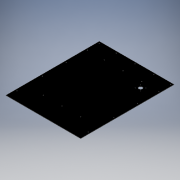
# Autodesk Inventor part: Side Cladding
Saved by Autodesk Inventor 2017.3 (Build 213256000, 256)
## iProperties
Created: 2018-10-13
Part Number: Side Cladding
Material: Aluminum 6061
Document SubType Name: Sheet Metal
Designer: Ax
Density: 2.7 g/cm^3
Sheet Metal Rule: Default_mm
Appearance: Anodized - Black
Author: Ax
Autodesk Inventor part; units mm, degrees
ref_plane "YZ Plane" through (0, 0, 0) normal (1, 0, 0) x (0, 1, 0)
ref_plane "XZ Plane" through (0, 0, 0) normal (0, 1, 0) x (-1, 0, 0)
ref_plane "XY Plane" through (0, 0, 0) normal (0, 0, 1) x (1, 0, 0)
sketch "Sketch1" plane through (0, 0, 0) normal (0, 0, 1) x (1, 0, 0)
  line L0 (-220, -275) -> (220, -275)
  line L1 (220, -275) -> (220, 275)
  line L2 (220, 275) -> (-220, 275)
  line L3 (-220, 275) -> (-220, -275)
  line L4 (-220, -275) -> (220, 275) construction
  line L5 (220, -275) -> (-220, 275) construction
  line L6 (-220, 265) -> (220, 265) construction
  line L7 (-210, 275) -> (-210, -275) construction
  line L8 (210, 275) -> (210, -275) construction
  line L9 (-220, -165) -> (220, -165) construction
  line L10 (-220, 195) -> (220, 195) construction
  circle A0 centre (-210, 265) radius 2.1
  circle A1 centre (-110, 265) radius 2.1
  circle A2 centre (110, 265) radius 2.1
  circle A3 centre (210, 265) radius 2.1
  circle A4 centre (110, 195) radius 2.1
  circle A5 centre (210, 195) radius 2.1
  circle A6 centre (-210, 195) radius 2.1
  circle A7 centre (-110, 195) radius 2.1
  line L11 (-110, 275) -> (-110, -275) construction
  line L12 (0, 0) -> (0, -275) construction
  line L13 (110, 275) -> (110, -275) construction
  circle A8 centre (-210, 70) radius 2.1
  circle A9 centre (110, -165) radius 2.1
  circle A10 centre (-110, -165) radius 2.1
  circle A11 centre (-210, -70) radius 2.1
  circle A12 centre (-210, -220) radius 2.1
  circle A13 centre (210, -220) radius 2.1
  circle A14 centre (210, -70) radius 2.1
  circle A15 centre (210, 70) radius 2.1
  line L14 (-210, 70) -> (210, 70) construction
  line L15 (-210, -70) -> (210, -70) construction
  line L16 (-210, 0) -> (210, 0) construction
  line L17 (-210, -220) -> (210, -220) construction
  line L18 (0, 275) -> (0, 0) construction
  circle A16 centre (0, 265) radius 2.1
  circle A17 centre (0, 195) radius 2.1
  circle A18 centre (0, -165) radius 2.1
  line L19 (118, 138) -> (160, 138) construction
  line L20 (160, 138) -> (160, 180) construction
  line L21 (160, 180) -> (118, 180) construction
  line L22 (118, 180) -> (118, 138) construction
  line L23 (118, 138) -> (160, 180) construction
  line L24 (160, 138) -> (118, 180) construction
  circle A19 centre (139, 159) radius 11
  line L25 (123.5, 143.5) -> (154.5, 143.5) construction
  line L26 (154.5, 143.5) -> (154.5, 174.5) construction
  line L27 (154.5, 174.5) -> (123.5, 174.5) construction
  line L28 (123.5, 174.5) -> (123.5, 143.5) construction
  line L29 (123.5, 143.5) -> (154.5, 174.5) construction
  line L30 (154.5, 143.5) -> (123.5, 174.5) construction
  circle A20 centre (123.5, 174.5) radius 1.7
  circle A21 centre (154.5, 174.5) radius 1.7
  circle A22 centre (154.5, 143.5) radius 1.7
  circle A23 centre (123.5, 143.5) radius 1.7
  dimension "d0" = 440
  dimension "d1" = 550
  dimension "d2" = 10
  dimension "d3" = 10
  dimension "d4" = 10
  dimension "d5" = 110
  dimension "d6" = 80
  dimension "d7" = 110
  dimension "d8" = 110
  dimension "d9" = 70
  dimension "d10" = 55
  dimension "d11" = 4.2
  dimension "d14" = 42
  dimension "d15" = 15
  dimension "d16" = 50
  dimension "d17" = 31
  dimension "d18" = 3.4
  dimension "d19" = 22
  measures "d0" distance of L1.end L2.end
  measures "d1" distance of L0.end L1.end
  measures "d2" distance of L2.end L6.start
  measures "d3" distance of L0.start L7.end
  measures "d4" distance of L0.end L8.end
  measures "d5" distance of L0.end L9.end
  measures "d6" distance of L10.end L1.end
  measures "d7" distance of L0.start L11.end
  measures "d8" distance of L13.end L0.end
  measures "d9" vertical distance of L12.start L14.start
  measures "d10" vertical distance of L0.end L17.end
  measures "d11" diameter of A7
  measures "d14" distance of L19.end L20.end
  measures "d15" vertical distance of A5.centre L20.end
  measures "d16" distance from line of L8 L20.end
  measures "d17" distance of L25.end L26.end
  measures "d18" diameter of A20
  measures "d19" diameter of A19
extrude "Plate3" add sketch "Sketch1" along normal blind 1.5
equation "\"BendRadius\" = Thickness"
equation "\"BendReliefWidth\" = Thickness"
equation "\"BendReliefDepth\" = 0.5 * Thickness"
equation "\"CornerReliefSize\" = 4 * Thickness"
equation "\"MinimumRemnant\" = 2 * Thickness"
equation "\"TransitionRadius\" = BendRadius"
equation "\"JacobiRadiusSize\" = BendRadius"
equation "\"GapSize\" = Thickness"
equation "\"d12\" = BendRadius"
equation "\"d13\" = BendRadius"
equation "\"d20\" = BendRadius"
equation "\"Thickness\" = 1.5"
body "Solid3"
